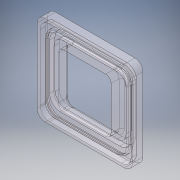
# Autodesk Inventor part: RAT WATER BOTTLE TRANSITION
Saved by Autodesk Inventor 2018.2 (Build 222227000, 227)
## iProperties
Created: 2017-06-29
Material: POLYCARBONATE, CLEAR
Vendor: HHMI: JRC - ID&F
Document SubType Name: Modeling
Designer: ROGERSR
Mass: 109.169 g
Surface Area: 352.846 cm^2
Volume: 90.974 cm^3
Density: 1.2 g/cm^3
Appearance: Polycarbonate (Clear)
RuleStatus: InUse
AfterDocSave0: file://Part Number Cleaner
DESIGN DEPARTMENT: HHMI: JRC - ID&F
ALTERED ITEM PART NUMBER: N/A
ALTERED ITEM VENDOR: N/A
ALTERED ITEM DESCRIPTION: N/A
Author: ROGERSR
Revision Number: 0
Autodesk Inventor part; units mm, degrees
ref_plane "YZ Plane" through (0, 0, 0) normal (1, 0, 0) x (0, 1, 0)
ref_plane "XZ Plane" through (0, 0, 0) normal (0, 1, 0) x (-1, 0, 0)
ref_plane "XY Plane" through (0, 0, 0) normal (0, 0, 1) x (1, 0, 0)
sketch "Sketch1" plane through (0, 0, 0) normal (0, 0, 1) x (1, 0, 0)
  line L0 (-60.325, -53.975) -> (60.325, -53.975)
  line L1 (60.325, -53.975) -> (60.325, 53.975)
  line L2 (60.325, 53.975) -> (-60.325, 53.975)
  line L3 (-60.325, 53.975) -> (-60.325, -53.975)
  line L4 (-60.325, -53.975) -> (60.325, 53.975) construction
  line L5 (60.325, -53.975) -> (-60.325, 53.975) construction
  point P0 (0, 0)
  dimension "d0" = 120.65
  dimension "d1" = 107.95
  constraints: 12 end point, 2 midpoint, 2 parallel, 1 horizontal, 1 perpendicular
  measures "d0" distance of L2.end L1.end
  measures "d1" distance of L1.end L0.end
extrude "Polycarbonate Plate" add sketch "Sketch1" along normal blind 12.7
sketch "Sketch2" plane through (0, 0, 12.7) normal (0, 0, 1) x (1, 0, 0)
  line L0 (-42.0687, -50.8) -> (44.2913, -50.8)
  line L1 (55.7212, -39.37) -> (55.7212, 39.37)
  line L2 (44.2912, 50.8) -> (-42.0687, 50.8)
  line L3 (-53.4987, 39.37) -> (-53.4987, -39.37)
  line L4 (-53.4987, -50.8) -> (55.7212, 50.8) construction
  line L5 (55.7212, -50.8) -> (-53.4987, 50.8) construction
  line L6 (-35.4647, 46.101) -> (37.6872, 46.101)
  line L7 (51.6573, 32.131) -> (51.6573, -32.131)
  line L8 (37.6874, -46.157) -> (-35.4649, -46.157)
  line L9 (-49.4347, -32.131) -> (-49.4347, 32.131)
  arc A0 (-51.9112, 50.8) -> (-53.4987, 49.2125) centre (-51.9112, 49.2125) ccw
  arc A1 (-35.4647, 46.101) -> (-49.4347, 32.131) centre (-35.4647, 32.131) ccw
  arc A2 (51.6573, 32.131) -> (37.6872, 46.101) centre (37.6872, 32.131) ccw
  arc A3 (37.6874, -46.157) -> (51.6573, -32.131) centre (37.6874, -32.187) ccw
  arc A4 (-49.4347, -32.131) -> (-35.4649, -46.157) centre (-35.4649, -32.187) ccw
  arc A5 (-42.0687, 50.8) -> (-53.4987, 39.37) centre (-42.0687, 39.37) ccw
  arc A6 (55.7212, 39.37) -> (44.2912, 50.8) centre (44.2912, 39.37) ccw
  arc A7 (44.2913, -50.8) -> (55.7212, -39.37) centre (44.2913, -39.37) ccw
  arc A8 (-53.4987, -39.37) -> (-42.0687, -50.8) centre (-42.0687, -39.37) ccw
  point P0 (1.1113, 0)
  dimension "d4" = 109.22
  dimension "d5" = 101.6
  dimension "d6" = 4.699
  dimension "d10" = 13.97
  dimension "d11" = 11.43
  dimension "d26" = 4.064
  dimension "d28" = 4.064
  constraints: 20 end point, 18 point on circle, 10 point on line, 9 centre point, 9 tangent, 6 equal radius, 2 midpoint, 2 parallel, 2 vertical, 1 horizontal
  measures "d4" distance of L5.end L4.end
  measures "d5" distance of L4.end L5.start
  measures "d6" distance between parallel lines of L2 L6
  measures "d10" radius of A1
  measures "d11" radius of A5
  measures "d26" distance between parallel lines of L9 L3
  measures "d28" distance between parallel lines of L1 L7
extrude "Lid Recess" cut sketch "Sketch2" against normal blind 6.35
sketch "Sketch3" plane through (0, 0, 0) normal (0, 0, -1) x (-1, 0, 0)
  line L0 (35.7188, -40.4812) -> (-35.7188, -40.4813)
  line L1 (-48.4187, -27.7813) -> (-48.4188, 27.7812)
  line L2 (-35.7188, 40.4812) -> (35.7187, 40.4812)
  line L3 (48.4188, 27.7812) -> (48.4188, -27.7812)
  line L4 (48.4188, -40.4812) -> (-48.4188, 40.4812) construction
  line L5 (-48.4188, -40.4813) -> (48.4188, 40.4813) construction
  line L6 (-43.3388, 23.9713) -> (-43.3388, -23.9713)
  line L7 (-31.9088, -35.4013) -> (31.9088, -35.4013)
  line L8 (43.3388, -23.9713) -> (43.3388, 23.9713)
  line L9 (31.9088, 35.4013) -> (-31.9088, 35.4013)
  arc A0 (-43.3388, -23.9713) -> (-31.9088, -35.4013) centre (-31.9088, -23.9713) ccw
  arc A1 (31.9088, -35.4013) -> (43.3388, -23.9713) centre (31.9088, -23.9713) ccw
  arc A2 (43.3388, 23.9713) -> (31.9088, 35.4013) centre (31.9088, 23.9713) ccw
  arc A3 (-31.9088, 35.4013) -> (-43.3388, 23.9713) centre (-31.9088, 23.9713) ccw
  arc A4 (-35.7188, 40.4812) -> (-48.4188, 27.7812) centre (-35.7188, 27.7812) ccw
  arc A5 (-48.4187, -27.7813) -> (-35.7188, -40.4813) centre (-35.7188, -27.7813) ccw
  arc A6 (35.7188, -40.4812) -> (48.4188, -27.7812) centre (35.7188, -27.7812) ccw
  arc A7 (48.4188, 27.7812) -> (35.7187, 40.4812) centre (35.7188, 27.7812) ccw
  point P0 (0, 0)
  dimension "d14" = 96.8375
  dimension "d15" = 80.9625
  dimension "d16" = 5.08
  dimension "d17" = 11.43
  dimension "d18" = 12.7
  constraints: 20 end point, 16 point on circle, 16 tangent, 8 centre point, 8 point on line, 6 equal radius, 4 parallel, 2 midpoint, 2 perpendicular, 1 horizontal, 3 other
  measures "d14" distance of L4.end L5.end
  measures "d15" distance of L5.start L4.end
  measures "d16" distance between parallel lines of L1 L6
  measures "d17" radius of A0
  measures "d18" radius of A4
fillet "Fillet1" radius 3.175 4 edges at (-60.325, 53.975, 6.35) (-60.325, -53.975, 6.35) (60.325, 53.975, 6.35) (60.325, -53.975, 6.35)
extrude "Small Recess" cut sketch "Sketch3" against normal blind 6.35
sketch "Sketch4" plane through (0, 0, 0) normal (0, 0, -1) x (-1, 0, 0)
  line L0 (-31.6778, 32.3024) -> (31.6778, 32.3024)
  line L1 (31.6778, 32.3024) -> (31.6778, -32.3024)
  line L2 (31.6778, -32.3024) -> (-31.6778, -32.3024)
  line L3 (-31.6778, -32.3024) -> (-31.6778, 32.3024)
  line L4 (-31.6778, 32.3024) -> (31.6778, -32.3024) construction
  line L5 (31.6778, 32.3024) -> (-31.6778, -32.3024) construction
  point P0 (0, 0)
  constraints: 12 end point, 2 midpoint, 2 parallel, 1 horizontal, 1 perpendicular
extrude "Inside Dimension" cut sketch "Sketch4" against normal through all
fillet "Fillet2" radius 6.35 4 edges at (-31.6778, 32.3024, 6.35) (31.6778, -32.3024, 6.35) (31.6778, 32.3024, 6.35) (-31.6778, -32.3024, 6.35)
fillet "Fillet3" radius 3.175 8 edges at (-29.8179, -30.4425, 0) (0, -32.3024, 0) (29.8179, -30.4425, 0) (31.6778, 0, 0) (29.8179, 30.4425, 0) (0, 32.3024, 0) (-29.8179, 30.4425, 0) (-31.6778, 0, 0)
sketch "Sketch5" plane through (0, 0, 12.7) normal (0, 0, 1) x (1, 0, 0)
  arc A0 (57.15, -53.975) -> (60.325, -50.8) centre (57.15, -50.8) ccw
  line L0 (60.325, -50.8) -> (60.325, 50.8)
  arc A1 (60.325, 50.8) -> (57.15, 53.975) centre (57.15, 50.8) ccw
  arc A2 (-57.15, 53.975) -> (-60.325, 50.8) centre (-57.15, 50.8) ccw
  line L1 (-60.325, 50.8) -> (-60.325, -50.8)
  arc A3 (-60.325, -50.8) -> (-57.15, -53.975) centre (-57.15, -50.8) ccw
  line L2 (57.15, 53.975) -> (57.15, -53.975)
  line L3 (-57.15, -53.975) -> (-57.15, 53.975)
  constraints: 8 end point, 8 point on circle, 7 centre point, 4 point on line
extrude "Extrusion5" cut sketch "Sketch5" against normal through all
fillet "Fillet4" radius 9.525 4 edges at (-57.15, 53.975, 6.35) (57.15, 53.975, 6.35) (57.15, -53.975, 6.35) (-57.15, -53.975, 6.35)
sketch "Sketch6" plane through (0, 0, 12.7) normal (0, 0, 1) x (1, 0, 0)
  arc A0 (-49.4347, -32.131) -> (-35.4649, -46.157) centre (-35.4649, -32.187) ccw
  line L0 (-35.4649, -46.157) -> (37.6874, -46.157)
  arc A1 (37.6874, -46.157) -> (51.6573, -32.131) centre (37.6874, -32.187) ccw
  line L1 (51.6573, -32.131) -> (51.6573, 32.131)
  arc A2 (51.6573, 32.131) -> (37.6872, 46.101) centre (37.6872, 32.131) ccw
  line L2 (37.6872, 46.101) -> (-35.4647, 46.101)
  arc A3 (-35.4647, 46.101) -> (-49.4347, 32.131) centre (-35.4647, 32.131) ccw
  line L3 (-49.4347, 32.131) -> (-49.4347, -32.131)
  arc A4 (-35.4647, 44.1873) -> (-47.521, 32.131) centre (-35.4647, 32.131) ccw
  line L4 (-35.4647, 44.1873) -> (37.6873, 44.1873)
  arc A5 (49.7435, 32.131) -> (37.6873, 44.1873) centre (37.6872, 32.131) ccw
  line L5 (49.7435, 32.131) -> (49.7435, -32.135)
  arc A6 (37.6874, -44.2432) -> (49.7435, -32.135) centre (37.6874, -32.187) ccw
  line L6 (37.6874, -44.2432) -> (-35.4649, -44.2432)
  arc A7 (-47.521, -32.135) -> (-35.4649, -44.2432) centre (-35.4649, -32.187) ccw
  line L7 (-47.521, -32.135) -> (-47.521, 32.131)
  constraints: 16 end point, 16 point on circle, 11 centre point, 4 horizontal, 4 vertical, 28 other
extrude "Extrusion6" cut sketch "Sketch6" against normal blind 3.175
equation "\"d28\" = d26"
body "Solid1"
